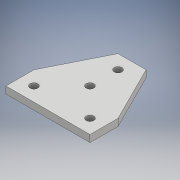
# Autodesk Inventor part: SupportCR-10-Mini
Saved by Autodesk Inventor 2018 (Build 220112000, 112)
## iProperties
Created: 2018-06-08
Part Number: SupportCR-10-Mini
Material: Generic
Document SubType Name: Modeling
Designer: JARVIS
Density: 1 g/cm^3
Appearance: Default
Author: JARVIS
Autodesk Inventor part; units mm, degrees
ref_plane "YZ Plane" through (0, 0, 0) normal (1, 0, 0) x (0, 1, 0)
ref_plane "XZ Plane" through (0, 0, 0) normal (0, 1, 0) x (-1, 0, 0)
ref_plane "XY Plane" through (0, 0, 0) normal (0, 0, 1) x (1, 0, 0)
sketch "Sketch1" plane through (0, 0, 0) normal (0, 0, 1) x (1, 0, 0)
  line L0 (-30, 0) -> (30, 0)
  line L1 (30, 0) -> (30, 20)
  line L2 (30, 20) -> (10, 60)
  line L3 (10, 60) -> (-10, 60)
  line L4 (-10, 60) -> (-30, 20)
  line L5 (-30, 20) -> (-30, 0)
  circle A0 centre (0, 50) radius 2.75
  circle A1 centre (0, 30) radius 2.75
  circle A2 centre (20, 10) radius 2.75
  circle A3 centre (-20, 10) radius 2.75
  point P0 (0, 0)
  point P1 (0, 0)
  point P2 (0, 60)
  dimension "d0" = 60
  dimension "d1" = 60
  dimension "d2" = 20
  dimension "d3" = 20
  dimension "d4" = 5.5
  dimension "d5" = 10
  dimension "d6" = 20
  dimension "d7" = 10
  dimension "d8" = 10
  dimension "d9" = 10
  constraints: 12 end point, 4 centre point, 3 equal radius, 3 vertical alignment, 2 coincident, 2 horizontal alignment, 2 midpoint, 2 perpendicular, 1 horizontal, 1 parallel
  measures "d0" distance of L0.start L0.end
  measures "d1" distance between parallel lines of L0 L3
  measures "d2" distance of L4.end L0.start
  measures "d3" distance of L2.end L3.end
  measures "d4" diameter of A0
  measures "d5" distance of point (0, 60) A0.centre
  measures "d6" distance of A1.centre A0.centre
  measures "d7" distance from line of L0 A2.centre
  measures "d8" distance from line of L1 A2.centre
  measures "d9" distance from line of L5 A3.centre
extrude "Extrusion1" add sketch "Sketch1" along normal blind 5
body "Solid1"
